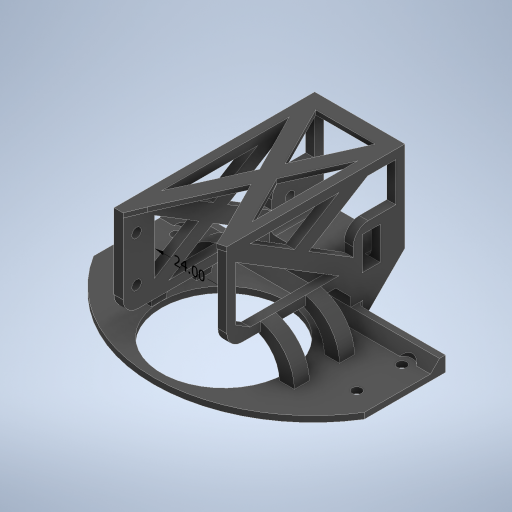
# Autodesk Inventor part: motor_setter
Saved by Autodesk Inventor 2024.1 (Build 281209000, 209)
## iProperties
Created: 2024-11-09
Part Number: motor_setter
Material: 一般
Document SubType Name: Modeling
Designer: hibik
Density: 1 g/cm^3
Appearance: 既定
Author: hibik
Autodesk Inventor part; units mm, degrees
ref_plane "YZ Plane" through (0, 0, 0) normal (1, 0, 0) x (0, 1, 0)
sketch "スケッチ1" plane through (0, 0, 0) normal (0, 0, 1) x (1, 0, 0)
  line L0 (30, -13) -> (-30, -13)
  line L1 (-30, -13) -> (-30, 13)
  line L2 (-30, 13) -> (30, 13)
  line L3 (30, 13) -> (30, -13)
  line L4 (30, -13) -> (-30, 13) construction
  line L5 (-30, -13) -> (30, 13) construction
  line L6 (45, -13) -> (-45, -13)
  line L7 (-45, -13) -> (-45, 13)
  line L8 (-45, 13) -> (45, 13)
  line L9 (45, 13) -> (45, -13)
  line L10 (45, -13) -> (-45, 13) construction
  line L11 (-45, -13) -> (45, 13) construction
  line L12 (-37.5, -13) -> (-37.5, 2.88938) construction
  line L13 (37.5, -13) -> (37.5, 2.88938) construction
  circle A0 centre (-37.5, -10) radius 1.6
  circle A1 centre (-37.5, -2) radius 1.6
  circle A2 centre (37.5, -10) radius 1.6
  circle A3 centre (37.5, -2) radius 1.6
  point P0 (0, 0)
  dimension "d0" = 60
  dimension "d1" = 26
  dimension "d2" = 90
  dimension "d3" = 7.5
  dimension "d4" = 7.5
  dimension "d5" = 3.2
  dimension "d6" = 3
  dimension "d7" = 8
  constraints: 28 end point, 6 point on line, 4 centre point, 4 midpoint, 4 parallel, 3 equal radius, 2 horizontal, 2 horizontal alignment, 2 perpendicular, 2 vertical, 1 collinear
  measures "d0" distance of L1.end L2.end
  measures "d1" distance of L0.end L1.end
  measures "d2" distance of L7.end L8.end
  measures "d3" distance between parallel lines of L1 L12
  measures "d4" distance between parallel lines of L3 L13
  measures "d5" diameter of A0
  measures "d6" distance from line of L6 A0.centre
  measures "d7" distance of A0.centre A1.centre
extrude "押し出し1" add sketch "スケッチ1" along normal blind 2
sketch "スケッチ2" plane through (0, 0, 0) normal (0, 0, -1) x (-1, 0, 0)
  line L0 (-12.5, 8) -> (11.5, 8)
  line L1 (11.5, 8) -> (11.5, 48)
  line L2 (11.5, 48) -> (-12.5, 48)
  line L3 (-12.5, 48) -> (-12.5, 8)
  line L4 (-45, 13) -> (45, 13) projected
  line L5 (11.5, 48) -> (14.5, 48)
  line L6 (14.5, 48) -> (14.5, 8)
  line L7 (14.5, 8) -> (11.5, 8)
  line L8 (11.5, 8) -> (11.5, 48)
  line L9 (-12.5, 48) -> (-15.5, 48)
  line L10 (-15.5, 48) -> (-15.5, 8)
  line L11 (-15.5, 8) -> (-12.5, 8)
  line L12 (-12.5, 8) -> (-12.5, 48)
  point P0 (0, 0)
  point P1 (-0.5, 48)
  point P2 (11.5, 13)
  point P3 (14.5, 13)
  point P4 (-15.5, 13)
  point P5 (-12.5, 13)
  dimension "d10" = 5
  dimension "d11" = 24
  dimension "d12" = 35
  dimension "d13" = 3
  dimension "d26" = 11.5
  constraints: 24 end point, 6 parallel, 3 horizontal, 3 perpendicular, 2 collinear, 1 midpoint, 1 point on line
  measures "d10" distance between parallel lines of L4 L0
  measures "d11" distance of L1.end L2.end
  measures "d12" distance between parallel lines of L4 L2
  measures "d13" distance of L1.end L5.end
  measures "d26" distance from line of point (0, 0) L1
extrude "押し出し2" add sketch "スケッチ2" against normal blind 53.7 contours L4 L10 L9 L3 | L1 L5 L6 L4
extrude "押し出し3" add sketch "スケッチ2" along normal blind 33.3 contours L4 L10 L9 L3 | L1 L5 L6 L4
sketch "スケッチ3" plane through (-14.5, 13, 53.7) normal (-1, 0, 0) x (0, 0, 1)
  circle A0 centre (-7.5, 30) radius 1.6
  circle A1 centre (-7.5, 15) radius 1.6
  circle A2 centre (-58.5, 15) radius 1.6
  line L0 (0, 35) -> (-87, 35) projected
  line L1 (-53.7, 0) -> (-53.7, -26) projected
  point P0 (-53.7, -13)
  dimension "d18" = 3.2
  dimension "d19" = 3.2
  dimension "d20" = 15
  dimension "d21" = 51
  dimension "d22" = 5
  dimension "d23" = 46.2
  constraints: 3 centre point, 1 equal radius, 1 horizontal alignment, 1 vertical alignment
  measures "d18" diameter of A0
  measures "d19" diameter of A1
  measures "d20" distance of A1.centre A0.centre
  measures "d21" distance of A2.centre A1.centre
  measures "d22" distance from line of L0 A0.centre
  measures "d23" distance from line of L1 A0.centre
extrude "押し出し4" cut sketch "スケッチ3" against normal up to surface (3 mm away)
sketch "スケッチ4" plane through (15.5, 13, 53.7) normal (1, 0, 0) x (0, 0, -1)
  line L0 (55.5, 19) -> (82.5, 19) projected
  line L1 (82.5, 19) -> (82.5, 35) projected
  line L2 (82.5, 35) -> (10.5, 35) projected
  line L3 (10.5, 35) -> (10.5, 10) projected
  line L4 (10.5, 10) -> (55.5, 10) projected
  line L5 (55.5, 10) -> (55.5, 19) projected
  line L6 (55.5, 19) -> (55.5, 0)
  line L7 (55.5, 19) -> (87, 19)
  line L8 (10.5, 10) -> (10.5, 0)
  line L9 (51.7, 0) -> (0, 0) projected
  line L10 (87, 35) -> (0, 35) projected
  line L11 (0, 0) -> (0, 35) projected
  line L12 (51.7, 0) -> (0, 0) projected
  line L13 (53.7, 0) -> (51.7, 0) projected
  line L14 (53.7, 0) -> (87, 0) projected
  line L15 (87, 35) -> (87, 0) projected
  point P0 (53.7, -13)
  point P1 (55.5, 0)
  point P2 (10.5, 35)
  constraints: 6 end point, 3 point on line, 2 vertical
extrude "押し出し5" cut sketch "スケッチ4" against normal up to surface (3 mm away) contours L0 L7 L15 L14 L6 L5 | L8 L9 L11 L10 L3
sketch "スケッチ6" plane through (-11.5, 13, 53.7) normal (1, 0, 0) x (0, 0, -1)
  line L0 (87, 35) -> (0, 35) projected
  line L1 (51.7, 0) -> (0, 0) projected
  circle A0 centre (7.5, 15) radius 1.6 projected
  circle A1 centre (58.5, 15) radius 1.6 projected
  circle A2 centre (7.5, 30) radius 1.6 projected
  line L2 (87, 35) -> (0, 35) projected
  line L3 (0, 0) -> (0, 35) projected
  line L4 (51.7, 0) -> (0, 0) projected
  line L5 (53.7, 0) -> (51.7, 0) projected
  line L6 (53.7, 0) -> (87, 0) projected
  line L7 (87, 35) -> (87, 0) projected
  line L8 (3, 35) -> (3, 0)
  point P0 (53.7, -13)
  point P1 (4.5, 35)
  dimension "d107" = 3
  constraints: 2 end point, 2 point on line, 1 perpendicular
  measures "d107" distance between parallel lines of L3 L8
extrude "押し出し6" cut sketch "スケッチ6" against normal through all contours L8 L1 L3 L0 | A0 | A1 | A2
sketch "スケッチ7" plane through (15.5, 13, 43.2) normal (1, 0, 0) x (0, 0, -1)
  line L0 (45, 19) -> (72, 19) projected
  line L1 (72, 19) -> (72, 35) projected
  line L2 (72, 35) -> (0, 35) projected
  line L3 (0, 35) -> (0, 10) projected
  line L4 (0, 10) -> (45, 10) projected
  line L5 (45, 10) -> (45, 19) projected
  line L6 (-7.5, 8) -> (76.5, 8)
  line L7 (-7.5, 35) -> (-7.5, 0) projected
  line L8 (76.5, 35) -> (76.5, 0) projected
  line L9 (-7.5, 35) -> (-7.5, 0) projected
  line L10 (41.2, 0) -> (-7.5, 0) projected
  line L11 (43.2, 0) -> (41.2, 0) projected
  line L12 (43.2, 0) -> (76.5, 0) projected
  line L13 (76.5, 35) -> (76.5, 0) projected
  line L14 (76.5, 35) -> (-7.5, 35) projected
  circle A0 centre (-3, 30) radius 1.6 projected
  circle A1 centre (48, 15) radius 1.6 projected
  circle A2 centre (-3, 15) radius 1.6 projected
  point P0 (43.2, -13)
  point P1 (-7.5, 0)
  dimension "d32" = 2
  constraints: 2 end point, 2 point on line, 1 horizontal
  measures "d32" distance between parallel lines of L4 L6
extrude "押し出し7" cut sketch "スケッチ7" against normal through all contours L8 L12 L11 L10 L7 L6
sketch "スケッチ8" plane through (15.5, 32, -33.3) normal (1, 0, 0) x (0, 0, -1)
  line L0 (-35.3, -45) -> (-35.3, -19)
  line L1 (-76.5, -11) -> (-31.5, -11)
  line L2 (-35.3, -11) -> (-35.3, -19.406688)
  line L3 (-35.3, -29) -> (-17.3, -11)
  line L4 (-84, -11) -> (0, -11)
  line L5 (-33.3, -19) -> (-35.3, -19)
  point P0 (-33.3, -32)
  point P1 (-35.3, -19)
  dimension "d35" = 45
  dimension "d36" = 10
  constraints: 4 end point, 4 point on line, 1 vertical
  measures "d35" angle of L4 L3
  measures "d36" distance from line of L5 L3.start
extrude "押し出し8" add sketch "スケッチ8" against normal up to surface (30 mm away)
sketch "スケッチ9" plane through (15.5, 32, -33.3) normal (1, 0, 0) x (0, 0, -1)
  line L0 (-35.3, -11) -> (-17.3, -11) projected
  line L1 (-17.3, -11) -> (-17.3, 16)
  line L2 (-84, 16) -> (0, 16) projected
  circle A0 centre (-79.5, -4) radius 1.6 projected
  circle A1 centre (-28.5, -4) radius 1.6 projected
  circle A2 centre (-79.5, 11) radius 1.6 projected
  line L3 (-84, -11) -> (-35.3, -11) projected
  line L4 (-35.3, -11) -> (-17.3, -11) projected
  line L5 (-17.3, -11) -> (0, -11) projected
  line L6 (0, 16) -> (0, -11) projected
  line L7 (0, 16) -> (-84, 16) projected
  line L8 (-84, 16) -> (-84, -11) projected
  point P0 (-33.3, -32)
  point P1 (-17.3, -11)
  point P2 (0, 16)
  point P3 (-87, 16)
  constraints: 2 end point, 1 point on line, 1 vertical
extrude "押し出し9" cut sketch "スケッチ9" against normal through all contours L1 L2 L6 L5
sketch "スケッチ10" plane through (15.5, 13, 2) normal (1, 0, 0) x (0, 0, -1)
  line L0 (9.8, 10) -> (9.8, 19) projected
  line L1 (18, 19) -> (18, 35) projected
  line L2 (18, 35) -> (-41.2, 35) projected
  line L3 (-41.2, 35) -> (-41.2, 8) projected
  line L4 (-41.2, 8) -> (0, 8) projected
  line L5 (0, 8) -> (0, 0) projected
  line L6 (2, 0) -> (0, 0) projected
  line L7 (2, -8) -> (2, 0) projected
  line L8 (2, -8) -> (18, 8) projected
  line L9 (18, 8) -> (3.8, 8) projected
  line L10 (3.8, 8) -> (3.8, 19) projected
  line L11 (3.8, 19) -> (18, 19) projected
  line L12 (18, 8) -> (18, 35) projected
  line L13 (18, 35) -> (-48.7, 35) projected
  line L14 (-48.7, 35) -> (-48.7, 8) projected
  line L15 (-48.7, 8) -> (0, 8) projected
  line L16 (0, 8) -> (18, 8) projected
  circle A0 centre (-44.2, 15) radius 1.6 projected
  circle A1 centre (6.8, 15) radius 1.6 projected
  circle A2 centre (-44.2, 30) radius 1.6 projected
  line L17 (9.8, 10) -> (9.8, 8)
  point P0 (2, -13)
  point P1 (9.8, 8)
  point P2 (18, 19)
  point P3 (9.8, 19)
  constraints: 2 end point, 1 perpendicular, 1 point on line
extrude "押し出し10" add sketch "スケッチ10" against normal up to surface (3 mm away) contours L0 L11 L12 L9 L17
fillet "フィレット1" radius 2 3 edges at (-11.5, 21, -7) (12.5, 21, 0.1) (12.5, 21, -11.9)
sketch "スケッチ11" plane through (0, 0, 0) normal (0, 0, -1) x (-1, 0, 0)
  circle A0 centre (37.5, -2) radius 1.6
  circle A1 centre (37.5, -10) radius 1.6
  circle A2 centre (-37.5, -10) radius 1.6
  circle A3 centre (-37.5, -2) radius 1.6
  line L0 (14.5, 13) -> (14.5, 5)
  line L1 (14.5, 5) -> (-15.5, 5)
  line L2 (-15.5, 5) -> (-15.5, 13)
  line L3 (-45, 13) -> (-15.5, 13)
  line L4 (-45, -13) -> (-45, 13)
  line L5 (45, -13) -> (-45, -13)
  line L6 (45, 13) -> (45, -13)
  line L7 (14.5, 13) -> (45, 13)
  line L8 (-45, 13) -> (-15.5, 13)
  line L9 (-17.5, 13) -> (17.5, 13)
  line L10 (17.5, 13) -> (17.5, 3)
  line L11 (17.5, 3) -> (-17.5, 3)
  line L12 (-17.5, 3) -> (-17.5, 13)
  line L13 (-32.5, 11) -> (32.5, 11)
  line L14 (32.5, 11) -> (32.5, -11)
  line L15 (32.5, -11) -> (-32.5, -11)
  line L16 (-32.5, -11) -> (-32.5, 11)
  line L17 (-33.182318, -10.268945) -> (-18.182318, 3.731055)
  line L18 (-18.182318, 3.731055) -> (-16.817682, 2.268945)
  line L19 (-16.817682, 2.268945) -> (-31.817682, -11.731055)
  line L20 (-31.817682, -11.731055) -> (-33.182318, -10.268945)
  line L21 (-33.182318, -10.268945) -> (-16.817682, 2.268945) construction
  line L22 (-18.182318, 3.731055) -> (-31.817682, -11.731055) construction
  line L23 (33.182318, -10.268945) -> (18.182318, 3.731055)
  line L24 (18.182318, 3.731055) -> (16.817682, 2.268945)
  line L25 (16.817682, 2.268945) -> (31.817682, -11.731055)
  line L26 (31.817682, -11.731055) -> (33.182318, -10.268945)
  line L27 (33.182318, -10.268945) -> (16.817682, 2.268945) construction
  line L28 (18.182318, 3.731055) -> (31.817682, -11.731055) construction
  line L29 (17.5, 3) -> (17.5, -11)
  line L30 (-17.5, 3) -> (-17.5, -11)
  line L31 (-17.902739, -10.084685) -> (32.097261, 11.915315)
  line L32 (32.097261, 11.915315) -> (32.902739, 10.084685)
  line L33 (32.902739, 10.084685) -> (-17.097261, -11.915315)
  line L34 (-17.097261, -11.915315) -> (-17.902739, -10.084685)
  line L35 (-17.902739, -10.084685) -> (32.902739, 10.084685) construction
  line L36 (32.097261, 11.915315) -> (-17.097261, -11.915315) construction
  line L37 (-32.097261, 11.915315) -> (17.902739, -10.084685)
  line L38 (17.902739, -10.084685) -> (17.097261, -11.915315)
  line L39 (17.097261, -11.915315) -> (-32.902739, 10.084685)
  line L40 (-32.902739, 10.084685) -> (-32.097261, 11.915315)
  line L41 (-32.097261, 11.915315) -> (17.097261, -11.915315) construction
  line L42 (17.902739, -10.084685) -> (-32.902739, 10.084685) construction
  line L43 (-18.182318, 3.731055) -> (-17.5, 4.367886)
  line L44 (-16.817682, 2.268945) -> (-16.034408, 3)
  line L45 (16.817682, 2.268945) -> (16.034408, 3)
  line L46 (18.182318, 3.731055) -> (17.5, 4.367886)
  line L47 (-17.902739, -10.084685) -> (-19.983, -11)
  line L48 (17.902739, -10.084685) -> (19.983, -11)
  line L49 (-43, 11) -> (-32.5, 11)
  line L50 (-32.5, 11) -> (-32.5, 3)
  line L51 (-32.5, 3) -> (-43, 3)
  line L52 (-43, 3) -> (-43, 11)
  line L53 (-32.902739, 10.084685) -> (-34.983, 11)
  line L54 (32.5, 11) -> (43, 11)
  line L55 (43, 11) -> (43, 3)
  line L56 (43, 3) -> (32.5, 3)
  line L57 (32.5, 3) -> (32.5, 11)
  line L58 (32.902739, 10.084685) -> (34.983, 11)
  circle A4 centre (-37.5, -2) radius 5
  circle A5 centre (37.5, -2) radius 5
  line L59 (-33.029464, 12.277251) -> (-38.432203, -1.638064)
  line L60 (-38.432203, -1.638064) -> (-36.567797, -2.361936)
  line L61 (-36.567797, -2.361936) -> (-31.165058, 11.553379)
  line L62 (-31.165058, 11.553379) -> (-33.029464, 12.277251)
  line L63 (-33.029464, 12.277251) -> (-36.567797, -2.361936) construction
  line L64 (-38.432203, -1.638064) -> (-31.165058, 11.553379) construction
  line L65 (31.165058, 11.553379) -> (36.567797, -2.361936)
  line L66 (36.567797, -2.361936) -> (38.432203, -1.638064)
  line L67 (38.432203, -1.638064) -> (33.029464, 12.277251)
  line L68 (33.029464, 12.277251) -> (31.165058, 11.553379)
  line L69 (31.165058, 11.553379) -> (38.432203, -1.638064) construction
  line L70 (36.567797, -2.361936) -> (33.029464, 12.277251) construction
  point P0 (0, 0)
  point P1 (0, -11)
  point P2 (0, 3)
  point P3 (-25, -4)
  point P4 (25, -4)
  point P5 (7.5, 0)
  point P6 (-6.25, 0)
  point P7 (-30.017, 11)
  point P8 (-17.5, 5.49252)
  point P9 (-17.5, 11)
  point P10 (17.5, 5.49252)
  point P11 (30.017, 11)
  point P12 (17.5, 11)
  point P13 (17.748232, 4.223446)
  point P14 (32.5, -9.632114)
  point P15 (32.5, 9.90748)
  point P16 (15.017, -11)
  point P17 (0, -4.39252)
  point P18 (-15.017, -11)
  point P19 (16.801182, 3)
  point P20 (2.483, -3.3)
  point P21 (31.034408, -11)
  point P22 (-11.835182, 3)
  point P23 (0, -2.20748)
  point P24 (11.835182, 3)
  point P25 (-2.483, -3.3)
  point P26 (-16.801182, 3)
  point P27 (-31.034408, -11)
  point P28 (-17.748232, 4.223446)
  point P29 (-32.5, 9.90748)
  point P30 (-32.5, -9.632114)
  point P31 (17.986959, 3.521742)
  point P32 (18.27214, 3.647222)
  point P33 (-18.27214, 3.647222)
  point P34 (-17.986959, 3.521742)
  point P35 (-16.280074, 2.770712)
  point P36 (16.280074, 2.770712)
  point P37 (-37.5, 3)
  point P38 (-32.5, -2)
  point P39 (32.5, -2)
  point P40 (37.5, 3)
  point P41 (-34.798631, 4.957658)
  point P42 (34.798631, 4.957658)
  point P43 (31.905631, 9.645958)
  point P44 (34.794681, 2.204908)
  point P45 (33.738048, 10.452221)
  point P46 (36.659087, 2.928779)
  point P47 (-34.794681, 2.204908)
  point P48 (-31.905631, 9.645958)
  point P49 (-36.659087, 2.928779)
  point P50 (-33.738048, 10.452221)
  dimension "d44" = 7.5
  dimension "d46" = 2
  dimension "d47" = 2
  dimension "d48" = 2
  dimension "d49" = 2
  dimension "d50" = 2
  dimension "d53" = 5
  dimension "d54" = 2
  dimension "d55" = 2
  constraints: 124 end point, 24 midpoint, 21 parallel, 14 perpendicular, 13 point on line, 6 collinear, 5 equal length, 4 coincident, 4 horizontal, 3 tangent, 2 centre point, 2 vertical alignment
  measures "d44" distance from line of L6 A0.centre
  measures "d46" distance between parallel lines of L2 L12
  measures "d47" distance between parallel lines of L3 L13
  measures "d48" distance between parallel lines of L5 L15
  measures "d49" distance between parallel lines of L1 L11
  measures "d50" distance between parallel lines of L17 L19
  measures "d53" distance from line of L51 A3.centre
  measures "d54" distance between parallel lines of L4 L52
  measures "d55" distance between parallel lines of L6 L55
extrude "押し出し11" cut sketch "スケッチ11" against normal through all contours A0 L65 L66 L67 | L67 L66 L65 A0 | L67 L56 A5 | A5 L14 L56 L65 | L56 L67 L58 L54 L55 | L14 L23 L33 L65 | L56 L14 L65 | L15 L48 L37 L29 L25 | L29 L37 L33 L45 L25 | L31 L10 L13 | L15 L33 L39 | L31 L37 L11 | L31 L30 L19 L44 L39 | L37 L13 L12 | L15 L19 L30 L31 L47 | L17 L16 L61 L39 | L16 L51 L61 | A4 L61 L51 L16 | L59 L51 L52 L49 L53 | L51 L59 A4 | L61 L60 L59 A3 | A3 L59 L60 L61 | A1 | A2
fillet "フィレット3" radius 2 2 edges at (15.5, 9, 0) (-14.5, 9, 0)
sketch "スケッチ12" plane through (-14.5, 48, 50.7) normal (0, 1, 0) x (1, 0, 0)
  line L0 (30, 66.7) -> (27, 66.7) projected
  line L1 (27, 7.5) -> (27, 66.7) projected
  line L2 (27, 7.5) -> (30, 7.5) projected
  line L3 (30, 66.7) -> (30, 7.5) projected
  line L4 (3, 66.7) -> (0, 66.7) projected
  line L5 (0, 0) -> (0, 66.7) projected
  line L6 (3, 66.7) -> (3, 0) projected
  line L7 (0, 0) -> (3, 0) projected
  point P0 (14.5, 50.7)
extrude "押し出し12" add sketch "スケッチ12" along normal blind 3
sketch "スケッチ13" plane through (-14.5, 51, 50.7) normal (0, 1, 0) x (1, 0, 0)
  line L0 (30, 66.7) -> (25, 66.7)
  line L1 (0, 52.7) -> (0, 66.7)
  line L2 (30, 66.7) -> (0, 66.7)
  line L3 (0, 66.7) -> (0, 61.7)
  line L4 (0, 61.7) -> (30, 61.7)
  line L5 (30, 61.7) -> (30, 66.7)
  line L6 (31.338219, 7.871728) -> (30, 12.689317)
  line L7 (30, 12.689317) -> (0, 4.355984)
  line L8 (0, 4.355984) -> (1.338219, -0.461606)
  line L9 (1.338219, -0.461606) -> (31.338219, 7.871728)
  line L10 (30, 7.5) -> (30, 66.7)
  line L11 (0, 66.7) -> (0, 0)
  line L12 (27.769992, 6.369928) -> (32.230008, 8.630072)
  line L13 (32.230008, 8.630072) -> (2.230008, 67.830072)
  line L14 (2.230008, 67.830072) -> (-2.230008, 65.569928)
  line L15 (-2.230008, 65.569928) -> (27.769992, 6.369928)
  line L16 (2.279996, -1.025485) -> (-2.279996, 1.025485)
  line L17 (-2.279996, 1.025485) -> (27.720004, 67.725485)
  line L18 (27.720004, 67.725485) -> (32.279996, 65.674515)
  line L19 (32.279996, 65.674515) -> (2.279996, -1.025485)
  line L20 (30, 7.5) -> (30, 66.7)
  line L21 (30, 66.7) -> (27, 66.7)
  line L22 (27, 66.7) -> (27, 7.5)
  line L23 (27, 7.5) -> (30, 7.5)
  line L24 (3, 0) -> (3, 66.7)
  line L25 (3, 66.7) -> (0, 66.7)
  line L26 (0, 66.7) -> (0, 0)
  line L27 (0, 0) -> (3, 0)
  point P0 (14.5, 50.7)
  point P1 (15.759161, 41.132544)
  point P2 (5.336464, 61.7)
  point P3 (25.009891, 61.7)
  point P4 (16.027971, 29.540848)
  point P5 (25.237934, 11.366521)
  point P6 (5.371555, 5.848083)
  point P7 (18.663693, 35.400935)
  point P8 (27, 53.935325)
  point P9 (3, 55.249378)
  point P10 (13.12344, 35.272457)
  point P11 (3, 12.764675)
  point P12 (27.19732, 7.5)
  point P13 (27, 7.889378)
  point P14 (27, 18.950622)
  point P15 (0, -3)
  dimension "d60" = 5
  constraints: 32 end point, 8 parallel, 5 point on line, 4 midpoint, 4 perpendicular, 3 equal length, 1 horizontal
  measures "d60" distance between parallel lines of L2 L4
extrude "押し出し13" add sketch "スケッチ13" against normal blind 1.5 contours L22 L17 L4 L13 L24 L2 L0 | L22 L4 L17 | L4 L22 L19 L13 L17 | L13 L4 L24 | L13 L17 L15 L24 L4 | L13 L19 L15 L17 | L13 L22 L7 L15 L19 | L15 L19 L7 L24 L17 | L22 L15 L7 | L15 L22 L23 L9 L24 L19 L7 | L19 L24 L7 | L15 L23 L22 | L9 L15 L23
chamfer "面取り1" distance 5 angle 45 2 edges at (14, 21, 2) (-13, 21, 2)
sketch "スケッチ14" plane through (15.5, 7, -2) normal (1, 0, 0) x (0, 0, -1)
  line L0 (-42.2, 41) -> (-3.2, 41)
  line L1 (-3.2, 41) -> (-3.2, 17)
  line L2 (-3.2, 17) -> (-42.2, 17)
  line L3 (-42.2, 17) -> (-42.2, 41)
  line L4 (-3.2, 41) -> (11, 41)
  line L5 (11, 41) -> (11, 28)
  line L6 (11, 28) -> (-3.2, 28)
  line L7 (-3.2, 28) -> (-3.2, 41)
  line L8 (-45.2, 14) -> (-45.2, 42.5)
  line L9 (14, 14) -> (14, 44)
  line L10 (-45.2, 44) -> (14, 44)
  line L11 (-45.2, 14) -> (-9, 14)
  line L12 (-0.2, 14) -> (-0.2, 25)
  line L13 (-0.2, 25) -> (5.8, 25)
  line L14 (-40.889756, 43.129146) -> (-43.510244, 38.870854)
  line L15 (-43.510244, 38.870854) -> (-4.510244, 14.870854)
  line L16 (-4.510244, 14.870854) -> (-1.889756, 19.129146)
  line L17 (-1.889756, 19.129146) -> (-40.889756, 43.129146)
  line L18 (-43.510244, 19.129146) -> (-40.889756, 14.870854)
  line L19 (-40.889756, 14.870854) -> (-1.889756, 38.870854)
  line L20 (-1.889756, 38.870854) -> (-4.510244, 43.129146)
  line L21 (-4.510244, 43.129146) -> (-43.510244, 19.129146)
  line L22 (-1.889756, 38.870854) -> (1.570105, 41)
  point P0 (-2, -7)
  point P1 (-22.7, 26.06455)
  point P2 (-37.429895, 17)
  point P3 (-7.970105, 17)
  point P4 (-17.929895, 29)
  point P5 (-3.2, 19.93545)
  point P6 (-3.2, 28)
  point P7 (-22.7, 31.93545)
  point P8 (-7.970105, 41)
  point P9 (-37.429895, 41)
  point P10 (-42.2, 19.93545)
  point P11 (-27.470105, 29)
  point P12 (-42.2, 38.06455)
  dimension "d66" = 3
  dimension "d67" = 3
  dimension "d68" = 3
  dimension "d69" = 3
  dimension "d70" = 3
  dimension "d71" = 3
  dimension "d72" = 5
  constraints: 34 end point, 8 parallel, 4 midpoint, 4 perpendicular, 2 horizontal, 1 collinear, 1 equal length, 1 point on line
  measures "d66" distance between parallel lines of L8 L3
  measures "d67" distance between parallel lines of L9 L5
  measures "d68" distance between parallel lines of L10 L0
  measures "d69" distance between parallel lines of L11 L2
  measures "d70" distance between parallel lines of L1 L12
  measures "d71" distance between parallel lines of L13 L6
  measures "d72" distance between parallel lines of L15 L17
extrude "押し出し14" cut sketch "スケッチ14" against normal through all contours L0 L21 L17 | L15 L21 L3 | L19 L1 L17 | L15 L2 L19 | L19 L22 L4 L5 L6 L1
fillet "フィレット4" radius 5 4 edges at (-13, 35, 1.2) (14, 35, 1.2) (14, 21, 43.2) (-13, 21, 50.7)
sketch "スケッチ15" plane through (0, 0, 2) normal (0, 0, 1) x (1, 0, 0)
  line L0 (30, 8) -> (45, 8)
  line L1 (-45, 13) -> (-45, -13)
  line L2 (-45, 8) -> (45, 8)
  line L3 (45, 8) -> (45, 10)
  line L4 (45, 10) -> (-45, 10)
  line L5 (-45, 10) -> (-45, 8)
  line L6 (45, -13) -> (45, 13)
  line L7 (-14.5, 16) -> (-11.5, 16)
  line L8 (-14.5, 16) -> (-14.5, 13)
  line L9 (-14.5, 13) -> (-45, 13)
  line L10 (-45, 13) -> (-45, -13)
  line L11 (-45, -13) -> (45, -13)
  line L12 (45, -13) -> (45, 13)
  line L13 (45, 13) -> (15.5, 13)
  line L14 (15.5, 16) -> (15.5, 13)
  line L15 (12.5, 23) -> (12.5, 16)
  arc A0 (10.5, 21) -> (12.5, 23) centre (10.5, 23) ccw
  line L16 (10.5, 21) -> (-9.5, 21)
  circle A1 centre (-37.5, -2) radius 1.6
  circle A2 centre (-37.5, -10) radius 1.6
  circle A3 centre (37.5, -10) radius 1.6
  circle A4 centre (37.5, -2) radius 1.6
  arc A5 (37.5, 3) -> (36.659087, 2.928779) centre (37.5, -2) ccw
  line L17 (36.659087, 2.928779) -> (33.738048, 10.452221)
  line L18 (33.738048, 10.452221) -> (34.983, 11)
  line L19 (34.983, 11) -> (43, 11)
  line L20 (43, 11) -> (43, 3)
  line L21 (43, 3) -> (37.5, 3)
  line L22 (-2.483, -3.3) -> (-19.983, -11)
  line L23 (-19.983, -11) -> (-31.034408, -11)
  line L24 (-31.034408, -11) -> (-16.280074, 2.770712)
  line L25 (-16.280074, 2.770712) -> (-2.483, -3.3)
  line L26 (17.5, 11) -> (30.017, 11)
  line L27 (30.017, 11) -> (17.5, 5.49252)
  line L28 (17.5, 5.49252) -> (17.5, 11)
  line L29 (31.034408, -11) -> (19.983, -11)
  line L30 (19.983, -11) -> (2.483, -3.3)
  line L31 (2.483, -3.3) -> (16.280074, 2.770712)
  line L32 (16.280074, 2.770712) -> (31.034408, -11)
  line L33 (-18.27214, 3.647222) -> (-32.5, -9.632114)
  line L34 (-32.5, -9.632114) -> (-32.5, -2)
  arc A6 (-32.5, -2) -> (-34.794681, 2.204908) centre (-37.5, -2) ccw
  line L35 (-34.794681, 2.204908) -> (-31.905631, 9.645958)
  line L36 (-31.905631, 9.645958) -> (-18.27214, 3.647222)
  line L37 (32.5, -2) -> (32.5, -9.632114)
  line L38 (32.5, -9.632114) -> (18.27214, 3.647222)
  line L39 (18.27214, 3.647222) -> (31.905631, 9.645958)
  line L40 (31.905631, 9.645958) -> (34.794681, 2.204908)
  arc A7 (34.794681, 2.204908) -> (32.5, -2) centre (37.5, -2) ccw
  line L41 (-11.835182, 3) -> (11.835182, 3)
  line L42 (11.835182, 3) -> (0, -2.20748)
  line L43 (0, -2.20748) -> (-11.835182, 3)
  line L44 (-17.5, 11) -> (-17.5, 5.49252)
  line L45 (-17.5, 5.49252) -> (-30.017, 11)
  line L46 (-30.017, 11) -> (-17.5, 11)
  line L47 (15.017, -11) -> (-15.017, -11)
  line L48 (-15.017, -11) -> (0, -4.39252)
  line L49 (0, -4.39252) -> (15.017, -11)
  line L50 (-34.983, 11) -> (-33.738048, 10.452221)
  line L51 (-33.738048, 10.452221) -> (-36.659087, 2.928779)
  arc A8 (-36.659087, 2.928779) -> (-37.5, 3) centre (-37.5, -2) ccw
  line L52 (-37.5, 3) -> (-43, 3)
  line L53 (-43, 3) -> (-43, 11)
  line L54 (-43, 11) -> (-34.983, 11)
  line L55 (12.5, 16) -> (15.5, 16)
  arc A9 (-11.5, 23) -> (-9.5, 21) centre (-9.5, 23) ccw
  line L56 (-11.5, 16) -> (-11.5, 23)
  point P0 (0, 0)
  point P1 (43, 10)
  point P2 (43, 8)
  point P3 (-17.5, 10)
  point P4 (-17.5, 8)
  point P5 (17.5, 8)
  point P6 (17.5, 10)
  point P7 (34.690143, 8)
  point P8 (33.913626, 10)
  point P9 (27.744273, 10)
  point P10 (23.198818, 8)
  point P11 (-33.913626, 10)
  point P12 (-34.690143, 8)
  point P13 (-23.198818, 8)
  point P14 (-27.744273, 10)
  point P15 (-43, 8)
  point P16 (-43, 10)
  dimension "d76" = 2
  constraints: 8 end point, 2 collinear, 2 parallel, 1 horizontal, 1 perpendicular, 1 point on line
  measures "d76" distance between parallel lines of L4 L0
extrude "押し出し15" add sketch "スケッチ15" along normal blind 50 contours L2 L39 L40 L0 | L40 L39 L2 L27 L4 L17 L0 | L17 L4 L20 L0 | L2 L28 L4 L27 | L20 L4 L3 L0 | L2 L44 L4 L28 | L2 L45 L4 L44 | L2 L36 L35 L51 L4 L45 | L2 L35 L36 | L1 L4 L53 L2 | L51 L2 L53 L4
sketch "スケッチ16" plane through (17.5, 10, 2) normal (0, 1, 0) x (1, 0, 0)
  circle A0 centre (-17.5, -26.7) radius 18.75 projected
  circle A1 centre (-17.5, -26.7) radius 20.75
  circle A2 centre (-55, -20) radius 1.35 projected
  circle A3 centre (-55, -5) radius 1.35 projected
  circle A4 centre (20, -20) radius 1.35 projected
  circle A5 centre (20, -5) radius 1.35 projected
  circle A6 centre (20, -5) radius 1.6
  circle A7 centre (20, -20) radius 1.6
  circle A8 centre (-55, -20) radius 1.6
  circle A9 centre (-55, -5) radius 1.6
  circle A10 centre (-17.5, -26.7) radius 23.3
  line L0 (27.5, -50) -> (-62.5, -50) projected
  arc A11 (-62.5, -25) -> (27.5, -25) centre (-17.5, 3) ccw
  line L1 (-62.5, 0) -> (-62.5, -50) projected
  line L2 (27.5, 0) -> (27.5, -50) projected
  point P0 (-17.5, 2)
  point P1 (-17.5, -50)
  dimension "d79" = 2
  dimension "d82" = 3.2
  constraints: 7 centre point, 6 coincident, 3 equal radius, 2 point on circle, 2 tangent, 2 other
  measures "d79" radial gap between concentric circles of A1 A0
  measures "d82" diameter of A6
extrude "押し出し16" cut sketch "スケッチ16" against normal through all contours A0 | A1 | A2 | A3 | A4 | A5 | A6 | A7 | A8 | A9 | A11 L2 L0 | L0 L1 A11
ref_plane "作業平面2" through (0, 0, 32) normal (0, 0, 1) x (1, 0, 0)
ref_plane "作業平面1" through (0, 0, 17) normal (0, 0, 1) x (1, 0, 0)
sketch "スケッチ17" plane through (0, 0, 32) normal (0, 0, 1) x (1, 0, 0)
  line L0 (-20.75, 10) -> (20.75, 10)
  line L1 (-20.75, 10) -> (-25.75, 10)
  line L2 (-14, 24) -> (-14.5, 24)
  line L3 (-14.5, 21) -> (-14.5, 26)
  line L4 (-14.5, 21) -> (-11.5, 21)
  arc A0 (-14.5, 24) -> (-25.75, 10) centre (-11.413889, 10) ccw
  arc A1 (-11.5, 21) -> (-20.75, 10) centre (-9.584459, 10) ccw
  line L5 (-25.75, 10) -> (-25.75, 8.904742)
  line L6 (-20.75, 10) -> (-20.75, 14.650329)
  point P0 (0, 0)
  point P1 (-11.5, 21)
  dimension "d104" = 5
  constraints: 8 end point, 4 point on circle, 2 centre point, 2 coincident, 2 tangent, 2 vertical, 1 horizontal, 1 parallel
  measures "d104" distance from line of L1.end L6
extrude "押し出し17" add sketch "スケッチ17" against normal blind 5
sketch "スケッチ18" plane through (0, 0, 17) normal (0, 0, 1) x (1, 0, 0)
  line L0 (-25.75, 10) -> (-20.75, 10)
  arc A0 (-11.5, 21) -> (-20.75, 10) centre (-9.584459, 10) ccw
  arc A1 (-14.5, 24) -> (-25.75, 10) centre (-11.413889, 10) ccw
  line L1 (-14.5, 21) -> (-14.5, 24)
  line L2 (-11.5, 21) -> (-14.5, 21)
  point P0 (0, 0)
extrude "押し出し18" add sketch "スケッチ18" against normal blind 5
ref_plane "作業平面3" through (0.5, 23, 2) normal (1, 0, 0) x (0, 0, -1)
mirror "ミラー1" about plane through (0.5, 23, 2) normal (1, 0, 0) of "押し出し17", "押し出し18"
sketch "スケッチ19" plane through (0, 0, 2) normal (0, 0, -1) x (-1, 0, 0)
  line L0 (-45, 13) -> (-17.5, 13)
  line L1 (16.5, 5) -> (-17.5, 5)
  line L2 (-17.5, 5.49252) -> (-17.5, 5)
  line L3 (-17.5, 5.49252) -> (-30.017, 11)
  line L4 (-30.017, 11) -> (-17.5, 11)
  line L5 (-17.5, 13) -> (-17.5, 11)
  line L6 (-45, 13) -> (-17.5, 13)
  line L7 (-45, -13) -> (-45, 13)
  line L8 (45, -13) -> (-45, -13)
  line L9 (45, 13) -> (45, -13)
  line L10 (16.5, 13) -> (45, 13)
  line L11 (16.5, 5) -> (16.5, 13)
  circle A0 centre (-37.5, -2) radius 1.6
  circle A1 centre (-37.5, -10) radius 1.6
  circle A2 centre (37.5, -10) radius 1.6
  circle A3 centre (37.5, -2) radius 1.6
  arc A4 (-36.659087, 2.928779) -> (-37.5, 3) centre (-37.5, -2) ccw
  line L12 (-37.5, 3) -> (-43, 3)
  line L13 (-43, 3) -> (-43, 11)
  line L14 (-43, 11) -> (-34.983, 11)
  line L15 (-34.983, 11) -> (-33.738048, 10.452221)
  line L16 (-33.738048, 10.452221) -> (-36.659087, 2.928779)
  line L17 (19.983, -11) -> (2.483, -3.3)
  line L18 (2.483, -3.3) -> (16.280074, 2.770712)
  line L19 (16.280074, 2.770712) -> (31.034408, -11)
  line L20 (31.034408, -11) -> (19.983, -11)
  line L21 (-19.983, -11) -> (-31.034408, -11)
  line L22 (-31.034408, -11) -> (-16.280074, 2.770712)
  line L23 (-16.280074, 2.770712) -> (-2.483, -3.3)
  line L24 (-2.483, -3.3) -> (-19.983, -11)
  line L25 (32.5, -9.632114) -> (18.27214, 3.647222)
  line L26 (18.27214, 3.647222) -> (31.905631, 9.645958)
  line L27 (31.905631, 9.645958) -> (34.794681, 2.204908)
  arc A5 (34.794681, 2.204908) -> (32.5, -2) centre (37.5, -2) ccw
  line L28 (32.5, -2) -> (32.5, -9.632114)
  line L29 (-32.5, -9.632114) -> (-32.5, -2)
  arc A6 (-32.5, -2) -> (-34.794681, 2.204908) centre (-37.5, -2) ccw
  line L30 (-34.794681, 2.204908) -> (-31.905631, 9.645958)
  line L31 (-31.905631, 9.645958) -> (-18.27214, 3.647222)
  line L32 (-18.27214, 3.647222) -> (-32.5, -9.632114)
  line L33 (-11.835182, 3) -> (11.835182, 3)
  line L34 (11.835182, 3) -> (0, -2.20748)
  line L35 (0, -2.20748) -> (-11.835182, 3)
  line L36 (17.5, 5.49252) -> (17.5, 11)
  line L37 (17.5, 11) -> (30.017, 11)
  line L38 (30.017, 11) -> (17.5, 5.49252)
  line L39 (15.017, -11) -> (-15.017, -11)
  line L40 (-15.017, -11) -> (0, -4.39252)
  line L41 (0, -4.39252) -> (15.017, -11)
  line L42 (33.738048, 10.452221) -> (34.983, 11)
  line L43 (34.983, 11) -> (43, 11)
  line L44 (43, 11) -> (43, 3)
  line L45 (43, 3) -> (37.5, 3)
  arc A7 (37.5, 3) -> (36.659087, 2.928779) centre (37.5, -2) ccw
  line L46 (36.659087, 2.928779) -> (33.738048, 10.452221)
  line L47 (-34.690143, 8) -> (-43, 8)
  line L48 (-28.164818, 8) -> (-32.544688, 8)
  line L49 (-17.5, 8) -> (-23.198818, 8)
  line L50 (23.198818, 8) -> (17.5, 8)
  line L51 (32.544688, 8) -> (28.164818, 8)
  line L52 (43, 8) -> (34.690143, 8)
  line L53 (-17.5, 11) -> (-17.5, 5.49252)
  point P0 (0, 0)
extrude "押し出し19" add sketch "スケッチ19" along normal up to surface (2 mm away) contours L53 L49 L3 L4 | L47 L13 L14 L15 L16 | L26 L27 L51 | L48 L30 L31 | L36 L37 L38 L50 | L42 L43 L44 L52 L46
chamfer "面取り2" distance 3 angle 45 1 edges at (0, 10, 2)
sketch "スケッチ20" plane through (0, 10, -1) normal (0, 1, 0) x (1, 0, 0)
  circle A0 centre (37.5, -8) radius 1.6 projected
  circle A1 centre (-37.5, -8) radius 1.6 projected
  circle A2 centre (37.5, -8) radius 3.5
  circle A3 centre (-37.5, -8) radius 3.5
  point P0 (0, -1)
  dimension "d100" = 7
  dimension "d101" = 7
  constraints: 2 centre point, 2 coincident
  measures "d100" diameter of A2
  measures "d101" diameter of A3
extrude "押し出し20" cut sketch "スケッチ20" along normal through all contours A0 | A1 | A2 | A3
sketch "スケッチ21" plane through (0, 0, 0) normal (0, 0, -1) x (-1, 0, 0)
  line L0 (-70, 8) -> (110, 8)
  line L1 (110, 8) -> (110, -30)
  line L2 (110, -30) -> (-70, -30)
  line L3 (-70, -30) -> (-70, 8)
  line L4 (-17.5, 8) -> (17.5, 8) projected
  point P0 (0, 0)
  constraints: 8 end point, 2 parallel, 1 collinear, 1 horizontal, 1 perpendicular
extrude "押し出し21" cut sketch "スケッチ21" against normal blind 10
sketch "スケッチ22" plane through (15.5, 7, -2) normal (1, 0, 0) x (0, 0, -1)
  line L0 (-27.470105, 29) -> (-22.7, 26.06455)
  line L1 (-27.470105, 29) -> (-42.2, 19.93545)
  line L2 (-37.429895, 17) -> (-22.7, 26.06455)
  line L3 (-42.2, 19.93545) -> (-37.429895, 17)
  point P0 (-2, -7)
  constraints: 4 end point
extrude "押し出し22" cut sketch "スケッチ22" against normal up to surface (3 mm away)
sketch "スケッチ23" plane through (-14.5, 51, 50.7) normal (0, 1, 0) x (1, 0, 0)
  line L0 (3, 12.764675) -> (3, 0)
  line L1 (30, 66.7) -> (0, 66.7)
  line L2 (0, 66.7) -> (0, 0)
  line L3 (0, 0) -> (3, 0)
  line L4 (3, 0) -> (30, 7.5)
  line L5 (30, 7.5) -> (30, 66.7)
  line L6 (27, 18.950622) -> (18.663693, 35.400935)
  line L7 (18.663693, 35.400935) -> (27, 53.935325)
  line L8 (27, 53.935325) -> (27, 18.950622)
  line L9 (15.759161, 41.132544) -> (5.336464, 61.7)
  line L10 (5.336464, 61.7) -> (25.009891, 61.7)
  line L11 (25.009891, 61.7) -> (15.759161, 41.132544)
  line L12 (16.027971, 29.540848) -> (25.237934, 11.366521)
  line L13 (25.237934, 11.366521) -> (5.371555, 5.848083)
  line L14 (5.371555, 5.848083) -> (16.027971, 29.540848)
  line L15 (3, 55.249378) -> (13.12344, 35.272457)
  line L16 (13.12344, 35.272457) -> (3, 12.764675)
  line L17 (3, 12.764675) -> (3, 55.249378)
  line L18 (3, 0) -> (5.371555, 5.848083)
  line L19 (27, 7.5) -> (27, 18.950622)
  line L20 (25.237934, 11.366521) -> (27.337097, 6.760305)
  point P0 (14.5, 50.7)
  constraints: 4 end point, 2 point on line
extrude "押し出し23" cut sketch "スケッチ23" against normal up to surface (1.5 mm away) contours L4 L18 L13 L20
equation "\"d4\" = d3"
equation "\"d18\" = d19"
equation "\"d47\" = d46"
equation "\"d48\" = d46"
equation "\"d49\" = d46"
equation "\"d54\" = d47"
equation "\"d55\" = d47"
equation "\"d67\" = d68"
equation "\"d68\" = d66"
equation "\"d69\" = d66"
equation "\"d71\" = d67"
